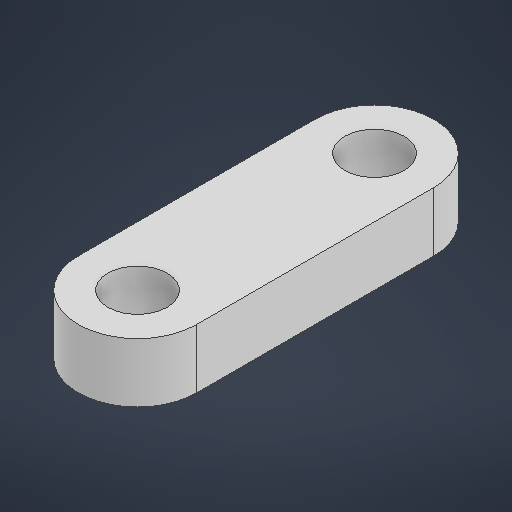
# Autodesk Inventor part: base
Saved by Autodesk Inventor 2027 (Build 310192060, 192F)
## iProperties
Created: 2026-08-01
Part Number: base
Material: Ogólny
Document SubType Name: Modeling
Designer: User
Density: 1 g/cm^3
Appearance: Domyślna
Author: User
Autodesk Inventor part; units mm, degrees
ref_plane "YZ Plane" through (0, 0, 0) normal (1, 0, 0) x (0, 1, 0)
ref_plane "XZ Plane" through (0, 0, 0) normal (0, 1, 0) x (-1, 0, 0)
ref_plane "XY Plane" through (0, 0, 0) normal (0, 0, 1) x (1, 0, 0)
sketch "Szkic1" plane through (0, 0, 0) normal (0, 1, 0) x (-1, 0, 0)
  line L0 (0, 0) -> (0, -8)
  circle A0 centre (0, 0) radius 1
  circle A1 centre (0, -8) radius 1
  line L1 (0, 0) -> (0, -8) construction
  line L2 (-2, 0) -> (-2, -8)
  line L3 (2, -8) -> (2, 0)
  arc A2 (2, 0) -> (-2, 0) centre (0, 0) ccw
  arc A3 (-2, -8) -> (2, -8) centre (0, -8) ccw
  point P0 (0, -4)
  dimension "d0" = 8
  dimension "d1" = 2
  dimension "d2" = 2
  dimension "d3" = 4
  constraints: 10 end point, 4 centre point, 4 point on circle, 4 tangent, 2 coincident, 2 equal length, 1 midpoint, 1 vertical
  measures "d0" distance of L0.start L0.end
  measures "d1" diameter of A0
  measures "d2" diameter of A1
  measures "d3" diameter of A3
extrude "Wyciągnięcie proste1" add sketch "Szkic1" against normal blind 2
